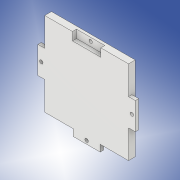
# Autodesk Inventor part: TC006
Saved by Autodesk Inventor 2017 SP1 (Build 210196100, 196)
## iProperties
Created: 2017-08-15
Part Number: TC006
Material: ABS Plastic
Document SubType Name: Modeling
Designer: Zach
Density: 1.06 g/cm^3
Appearance: CR White
Author: Zach
Autodesk Inventor part; units mm, degrees
ref_plane "YZ Plane" through (0, 0, 0) normal (1, 0, 0) x (0, 1, 0)
ref_plane "XZ Plane" through (0, 0, 0) normal (0, 1, 0) x (-1, 0, 0)
ref_plane "XY Plane" through (0, 0, 0) normal (0, 0, 1) x (1, 0, 0)
sketch "Sketch1" plane through (0, 0, 0) normal (0, 0, 1) x (1, 0, 0)
  line L0 (0, 0) -> (124, 0)
  line L1 (124, 0) -> (124, 124)
  line L2 (124, 124) -> (0, 124)
  line L3 (0, 124) -> (0, 0)
  dimension "d0" = 124
  dimension "d1" = 124
  constraints: 8 end point, 2 parallel, 1 horizontal, 1 perpendicular
  measures "d0" distance of L2.end L1.end
  measures "d1" distance of L1.end L0.end
extrude "Extrusion1" add sketch "Sketch1" along normal blind 10
sketch "Sketch2" plane through (0, 0, 10) normal (0, 0, 1) x (1, 0, 0)
  line L0 (0, 124) -> (0, 0) projected
  line L1 (0, 82) -> (-10, 82)
  line L2 (-10, 82) -> (-10, 42)
  line L3 (-10, 42) -> (0, 42)
  line L4 (0, 42) -> (0, 82)
  line L5 (0, 0) -> (124, 0) projected
  line L6 (42, 0) -> (82, 0)
  line L7 (82, 0) -> (82, -10)
  line L8 (82, -10) -> (42, -10)
  line L9 (42, -10) -> (42, 0)
  circle A0 centre (-5, 62) radius 2.5
  circle A1 centre (62, -5) radius 2.5
  point P0 (42, -5)
  point P1 (-10, 62)
  point P2 (-5, 82)
  point P3 (62, -10)
  point P4 (62, 0)
  point P5 (62, 0)
  point P6 (0, 62)
  dimension "d4" = 10
  dimension "d5" = 40
  dimension "d6" = 40
  dimension "d7" = 10
  dimension "d8" = 5
  dimension "d9" = 5
  constraints: 16 end point, 7 midpoint, 4 parallel, 4 vertical alignment, 3 horizontal alignment, 2 centre point, 2 horizontal, 2 perpendicular, 2 point on line
  measures "d4" distance of L3.end L2.end
  measures "d5" distance of L2.end L1.end
  measures "d6" distance of L7.end L8.end
  measures "d7" distance of L6.end L7.end
  measures "d8" diameter of A0
  measures "d9" diameter of A1
extrude "Extrusion2" add sketch "Sketch2" against normal blind 5
sketch "Sketch3" plane through (0, 0, 10) normal (0, 0, 1) x (1, 0, 0)
  line L0 (124, 124) -> (0, 124) projected
  line L1 (41, 124) -> (83, 124)
  line L2 (83, 124) -> (83, 112)
  line L3 (83, 112) -> (41, 112)
  line L4 (41, 112) -> (41, 124)
  point P0 (0, 0)
  point P1 (62, 112)
  point P2 (62, 124)
  dimension "d12" = 42
  dimension "d13" = 12
  constraints: 8 end point, 2 midpoint, 2 parallel, 1 horizontal, 1 perpendicular, 1 point on line, 1 vertical alignment
  measures "d12" distance of L2.end L3.end
  measures "d13" distance of L1.end L2.end
extrude "Extrusion3" cut sketch "Sketch3" against normal blind 6
sketch "Sketch4" plane through (0, 0, 4) normal (0, 0, 1) x (1, 0, 0)
  line L0 (41, 124) -> (83, 124) construction
  line L1 (41, 112) -> (41, 124) construction
  line L2 (83, 112) -> (41, 112) construction
  line L3 (83, 124) -> (83, 112) construction
  circle A0 centre (62, 119) radius 2.5
  point P0 (0, 0)
  point P1 (62, 124)
  dimension "d16" = 5
  dimension "d17" = 5
  constraints: 1 centre point, 1 midpoint, 1 vertical alignment
  measures "d16" diameter of A0
  measures "d17" distance from line of L0 A0.centre
extrude "Extrusion4" cut sketch "Sketch4" against normal through all
sketch "Sketch5" plane through (0, 0, 10) normal (0, 0, 1) x (1, 0, 0)
  line L0 (124, 0) -> (124, 124) projected
  line L1 (124, 82) -> (134, 82)
  line L2 (134, 82) -> (134, 42)
  line L3 (134, 42) -> (124, 42)
  line L4 (124, 42) -> (124, 82)
  circle A0 centre (129, 62) radius 2.5
  point P0 (0, 0)
  point P1 (134, 62)
  point P2 (124, 62)
  point P3 (124, 62)
  point P4 (129, 82)
  dimension "d20" = 10
  dimension "d21" = 40
  dimension "d22" = 5
  constraints: 8 end point, 4 midpoint, 3 horizontal alignment, 2 parallel, 1 centre point, 1 horizontal, 1 perpendicular, 1 point on line, 1 vertical alignment
  measures "d20" distance of L2.end L3.end
  measures "d21" distance of L1.end L2.end
  measures "d22" diameter of A0
extrude "Extrusion5" add sketch "Sketch5" against normal blind 5
body "Solid1"
